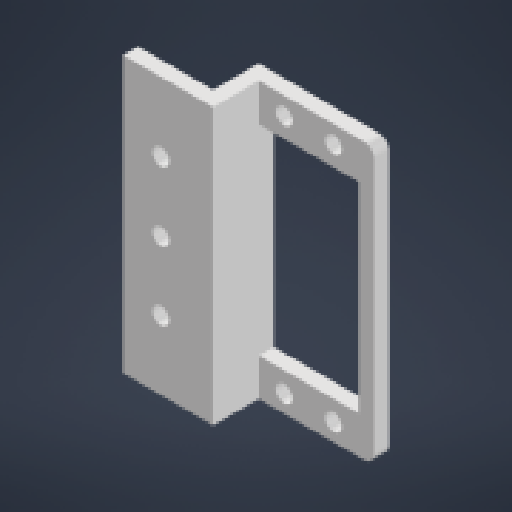
# Autodesk Inventor part: ServoMount
Saved by Autodesk Inventor 2023 (Build 270158000, 158)
## iProperties
Created: 2022-12-08
Part Number: ServoMount
Material: Generic
Document SubType Name: Modeling
Designer: izack
Density: 1 g/cm^3
Appearance: Default
Author: izack
Autodesk Inventor part; units mm, degrees
ref_plane "YZ Plane" through (0, 0, 0) normal (1, 0, 0) x (0, 1, 0)
ref_plane "XZ Plane" through (0, 0, 0) normal (0, 1, 0) x (-1, 0, 0)
sketch "Sketch1" plane through (0, 0, 0) normal (0, 0, 1) x (1, 0, 0)
  line L0 (0, -1000) -> (0, -848) construction
  line L1 (-15, -848) -> (-15, -1000) construction
  line L2 (-15, -963.9285) -> (0, -963.9285)
  line L3 (0, -963.9285) -> (0, -908.9285)
  line L4 (0, -908.9285) -> (-15, -908.9285)
  line L5 (-15, -908.9285) -> (-15, -963.9285)
  line L6 (0, -963.9285) -> (3, -963.9285)
  line L7 (3, -963.9285) -> (3, -908.9285)
  line L8 (3, -908.9285) -> (0, -908.9285)
  line L9 (0, -908.9285) -> (0, -963.9285)
  line L10 (-7.5, -908.9285) -> (-7.5, -963.9285) construction
  circle A0 centre (-7.5, -922.6785) radius 1.7
  circle A1 centre (-7.5, -936.4285) radius 1.7
  circle A2 centre (-7.5, -950.1785) radius 1.7
  line L11 (-15, -936.4285) -> (3, -936.4285) construction
  point P0 (0, 0)
  dimension "d6" = 55
  dimension "d7" = 3
  dimension "d22" = 3.4
  dimension "d23" = 3.4
  dimension "d24" = 3.4
  dimension "d25" = 13.75
  dimension "d26" = 13.75
  constraints: 20 end point, 5 midpoint, 5 point on line, 4 parallel, 3 centre point, 2 horizontal, 2 perpendicular
  measures "d6" distance of L3.end L2.end
  measures "d7" distance of L8.end L7.end
  measures "d22" diameter of A0
  measures "d23" diameter of A1
  measures "d24" diameter of A2
  measures "d25" distance of A2.centre A1.centre
  measures "d26" distance of A0.centre A1.centre
extrude "Extrusion1" add sketch "Sketch1" along normal blind 3
sketch "Sketch2" plane through (0, 0, 0) normal (0, 0, -1) x (-1, 0, 0)
  line L0 (-3, -963.9285) -> (-3, -908.9285) projected
  line L1 (-3, -908.9285) -> (15, -908.9285) projected
  line L2 (-3, -963.9285) -> (0, -963.9285)
  line L3 (0, -963.9285) -> (0, -908.9285)
  line L4 (0, -908.9285) -> (-3, -908.9285)
  line L5 (-3, -908.9285) -> (-3, -963.9285)
  point P0 (0, 0)
  constraints: 8 end point, 2 parallel, 1 horizontal, 1 perpendicular, 1 point on line
ref_plane "Work Plane1" through (54.1997, -954.1849, -9.0948) normal (0, 0, 1) x (0.9638, -0.2666, 0)
extrude "Extrusion2" add sketch "Sketch2" along normal up to surface (9.0948 mm away)
sketch "Sketch3" plane through (3, -963.9285, -9.0948) normal (0, 0, -1) x (-1, 0, 0)
  line L0 (0, 0) -> (0, 55) projected
  line L1 (0, 27.5) -> (-10, 27.5) construction
  line L2 (-20, 7.5) -> (0, 7.5)
  line L3 (0, 7.5) -> (0, 47.5)
  line L4 (0, 47.5) -> (-20, 47.5)
  line L5 (-20, 47.5) -> (-20, 7.5)
  line L6 (-20, 7.5) -> (0, 47.5) construction
  line L7 (0, 7.5) -> (-20, 47.5) construction
  line L8 (-14.95, 3.5) -> (-5.05, 3.5) construction
  line L9 (-5.05, 3.5) -> (-5.05, 51.5) construction
  line L10 (-5.05, 51.5) -> (-14.95, 51.5) construction
  line L11 (-14.95, 51.5) -> (-14.95, 3.5) construction
  line L12 (-14.95, 3.5) -> (-5.05, 51.5) construction
  line L13 (-5.05, 3.5) -> (-14.95, 51.5) construction
  circle A0 centre (-14.95, 3.5) radius 1.7
  line L14 (-10, 3.5) -> (-10, 51.5) construction
  circle A1 centre (-14.95, 51.5) radius 1.7
  circle A2 centre (-5.05, 3.5) radius 1.7
  circle A3 centre (-5.05, 51.5) radius 1.7
  line L15 (3, 0) -> (-21, 0)
  line L16 (-23, 2) -> (-23, 53)
  line L17 (-21, 55) -> (3, 55)
  line L18 (3, 55) -> (3, 0)
  line L19 (3, 0) -> (-23, 55) construction
  line L20 (-23, 0) -> (3, 55) construction
  arc A4 (-23, 2) -> (-21, 0) centre (-21, 2) ccw
  arc A5 (-21, 55) -> (-23, 53) centre (-21, 53) ccw
  point P0 (3, 963.9285)
  point P1 (0, 7.5)
  dimension "d12" = 10
  dimension "d13" = 40
  dimension "d14" = 9.9
  dimension "d15" = 48
  dimension "d16" = 3.4
  dimension "d17" = 26
  dimension "d18" = 55
  dimension "d19" = 2
  constraints: 40 end point, 9 midpoint, 6 centre point, 6 parallel, 5 point on line, 4 horizontal, 4 point on circle, 4 tangent, 3 perpendicular, 3 symmetric about line, 1 coincident, 1 equal radius, 3 other
  measures "d12" distance of L1.start L1.end
  measures "d13" distance of L3.end L2.end
  measures "d14" distance of L10.end L9.end
  measures "d15" distance of L9.end L8.end
  measures "d16" diameter of A0
  measures "d17" distance of L19.end L17.end
  measures "d18" distance of L20.start L19.end
  measures "d19" radius of A4
extrude "Extrusion3" add sketch "Sketch3" against normal blind 3 contours L15 A4 L16 A5 L17 L0 L4 L5 L2 | L0 L17 L18 L15
body "Solid1"
